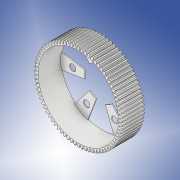
# Autodesk Inventor part: Flexspline
Saved by Autodesk Inventor 2017 SP1 (Build 210196100, 196)
## iProperties
Created: 2017-07-11
Part Number: Flexspline
Material: ABS Plastic
Document SubType Name: Modeling
Designer: zallen
Density: 1.06 g/cm^3
Appearance: CR White
Author: zallen
Autodesk Inventor part; units mm, degrees
ref_plane "YZ Plane" through (0, 0, 0) normal (1, 0, 0) x (0, 1, 0)
ref_plane "XZ Plane" through (0, 0, 0) normal (0, 1, 0) x (-1, 0, 0)
ref_plane "XY Plane" through (0, 0, 0) normal (0, 0, 1) x (1, 0, 0)
sketch "Sketch1" plane through (0, 0, 0) normal (0, 0, 1) x (1, 0, 0)
  circle A0 centre (0, 0) radius 44
  circle A1 centre (0, 0) radius 47 construction
  line L0 (0, 0) -> (52.2063, 0) construction
  arc A2 (46.9962, 0.6) -> (43.9777, 1.4) centre (41.6649, -13.4206) ccw
  arc A3 (46.9962, -0.6) -> (46.9962, 0.6) centre (27.0052, 0) ccw
  arc A4 (43.9777, -1.4) -> (46.9962, -0.6) centre (41.6649, 13.4206) ccw
  arc A5 (43.9777, -1.4) -> (43.9777, 1.4) centre (0, 0) ccw
  arc A6 (46.7861, 4.4789) -> (43.7119, 5.0269) centre (42.6309, -9.9341) ccw
  arc A7 (43.9431, 2.2364) -> (46.8852, 3.283) centre (40.4144, 16.8155) ccw
  arc A8 (46.8852, 3.283) -> (46.7861, 4.4789) centre (26.9129, 2.2301) ccw
  circle A9 centre (0, 0) radius 44
  arc A10 (43.9431, 2.2364) -> (43.7119, 5.0269) centre (0, 0) ccw
  arc A11 (46.2564, 8.3271) -> (43.1475, 8.6194) centre (43.3057, -6.3798) ccw
  arc A12 (43.6084, 5.8576) -> (46.454, 7.1435) centre (38.8877, 20.0954) ccw
  arc A13 (46.454, 7.1435) -> (46.2564, 8.3271) centre (26.6369, 4.4449) ccw
  circle A14 centre (0, 0) radius 44
  arc A15 (43.6084, 5.8576) -> (43.1475, 8.6194) centre (0, 0) ccw
  arc A16 (45.4108, 12.1185) -> (42.2883, 12.1531) centre (43.6846, -2.7818) ccw
  arc A17 (42.9757, 9.4387) -> (45.7054, 10.9552) centre (37.0954, 23.2381) ccw
  arc A18 (45.7054, 10.9552) -> (45.4108, 12.1185) centre (26.1788, 6.6294) ccw
  circle A19 centre (0, 0) radius 44
  arc A20 (42.9757, 9.4387) -> (42.2883, 12.1531) centre (0, 0) ccw
  arc A21 (44.255, 15.8271) -> (41.1403, 15.6037) centre (43.7651, 0.8351) ccw
  arc A22 (42.0495, 12.9554) -> (44.6446, 14.6921) centre (35.0498, 26.222) ccw
  arc A23 (44.6446, 14.6921) -> (44.255, 15.8271) centre (25.542, 8.7686) ccw
  circle A24 centre (0, 0) radius 44
  arc A25 (42.0495, 12.9554) -> (41.1403, 15.6037) centre (0, 0) ccw
  arc A26 (42.7968, 19.4276) -> (39.7113, 18.9477) centre (43.5467, 4.4464) ccw
  arc A27 (40.836, 16.3836) -> (43.2789, 18.3287) centre (32.7646, 29.0269) ccw
  arc A28 (43.2789, 18.3287) -> (42.7968, 19.4276) centre (24.7306, 10.8479) ccw
  circle A29 centre (0, 0) radius 44
  arc A30 (40.836, 16.3836) -> (39.7113, 18.9477) centre (0, 0) ccw
  arc A31 (41.0463, 22.8954) -> (38.0109, 22.1623) centre (43.0307, 8.0272) ccw
  arc A32 (39.3436, 19.6998) -> (41.6175, 21.84) centre (30.2557, 31.6334) ccw
  arc A33 (41.6175, 21.84) -> (41.0463, 22.8954) centre (23.7503, 12.853) ccw
  circle A34 centre (0, 0) radius 44
  arc A35 (39.3436, 19.6998) -> (38.0109, 22.1623) centre (0, 0) ccw
  arc A36 (39.0154, 26.2068) -> (36.0509, 25.2256) centre (42.2209, 11.5533) ccw
  arc A37 (37.5824, 22.8815) -> (39.6718, 25.2022) centre (27.5401, 34.0239) ccw
  arc A38 (39.6718, 25.2022) -> (39.0154, 26.2068) centre (22.6078, 14.7704) ccw
  circle A39 centre (0, 0) radius 44
  arc A40 (37.5824, 22.8815) -> (36.0509, 25.2256) centre (0, 0) ccw
  arc A41 (36.7181, 29.3391) -> (33.8447, 28.1165) centre (41.1226, 15.0004) ccw
  arc A42 (35.5645, 25.9069) -> (37.4551, 28.3922) centre (24.6364, 36.1819) ccw
  arc A43 (37.4551, 28.3922) -> (36.7181, 29.3391) centre (21.3109, 16.5869) ccw
  circle A44 centre (0, 0) radius 44
  arc A45 (35.5645, 25.9069) -> (33.8447, 28.1165) centre (0, 0) ccw
  arc A46 (34.1698, 32.2711) -> (31.4073, 30.8153) centre (39.7434, 18.345) ccw
  arc A47 (33.3037, 28.7553) -> (34.9826, 31.3882) centre (21.5644, 38.0928) ccw
  arc A48 (34.9826, 31.3882) -> (34.1698, 32.2711) centre (19.8684, 18.2901) ccw
  circle A49 centre (0, 0) radius 44
  arc A50 (33.3037, 28.7553) -> (31.4073, 30.8153) centre (0, 0) ccw
  arc A51 (31.3882, 34.9826) -> (28.7553, 33.3037) centre (38.0928, 21.5644) ccw
  arc A52 (30.8153, 31.4073) -> (32.2711, 34.1698) centre (18.345, 39.7434) ccw
  arc A53 (32.2711, 34.1698) -> (31.3882, 34.9826) centre (18.2901, 19.8684) ccw
  circle A54 centre (0, 0) radius 44
  arc A55 (30.8153, 31.4073) -> (28.7553, 33.3037) centre (0, 0) ccw
  arc A56 (28.3922, 37.4551) -> (25.9069, 35.5645) centre (36.1819, 24.6364) ccw
  arc A57 (28.1165, 33.8447) -> (29.3391, 36.7181) centre (15.0004, 41.1226) ccw
  arc A58 (29.3391, 36.7181) -> (28.3922, 37.4551) centre (16.5869, 21.3109) ccw
  circle A59 centre (0, 0) radius 44
  arc A60 (28.1165, 33.8447) -> (25.9069, 35.5645) centre (0, 0) ccw
  arc A61 (25.2022, 39.6718) -> (22.8815, 37.5824) centre (34.0239, 27.5401) ccw
  arc A62 (25.2256, 36.0509) -> (26.2068, 39.0154) centre (11.5533, 42.2209) ccw
  arc A63 (26.2068, 39.0154) -> (25.2022, 39.6718) centre (14.7704, 22.6078) ccw
  circle A64 centre (0, 0) radius 44
  arc A65 (25.2256, 36.0509) -> (22.8815, 37.5824) centre (0, 0) ccw
  arc A66 (21.84, 41.6175) -> (19.6998, 39.3436) centre (31.6334, 30.2557) ccw
  arc A67 (22.1623, 38.0109) -> (22.8954, 41.0463) centre (8.0272, 43.0307) ccw
  arc A68 (22.8954, 41.0463) -> (21.84, 41.6175) centre (12.853, 23.7503) ccw
  circle A69 centre (0, 0) radius 44
  arc A70 (22.1623, 38.0109) -> (19.6998, 39.3436) centre (0, 0) ccw
  arc A71 (18.3287, 43.2789) -> (16.3836, 40.836) centre (29.0269, 32.7646) ccw
  arc A72 (18.9477, 39.7113) -> (19.4276, 42.7968) centre (4.4464, 43.5467) ccw
  arc A73 (19.4276, 42.7968) -> (18.3287, 43.2789) centre (10.8479, 24.7306) ccw
  circle A74 centre (0, 0) radius 44
  arc A75 (18.9477, 39.7113) -> (16.3836, 40.836) centre (0, 0) ccw
  arc A76 (14.6921, 44.6446) -> (12.9554, 42.0495) centre (26.222, 35.0498) ccw
  arc A77 (15.6037, 41.1403) -> (15.8271, 44.255) centre (0.8351, 43.7651) ccw
  arc A78 (15.8271, 44.255) -> (14.6921, 44.6446) centre (8.7686, 25.542) ccw
  circle A79 centre (0, 0) radius 44
  arc A80 (15.6037, 41.1403) -> (12.9554, 42.0495) centre (0, 0) ccw
  arc A81 (10.9552, 45.7054) -> (9.4387, 42.9757) centre (23.2381, 37.0954) ccw
  arc A82 (12.1531, 42.2883) -> (12.1185, 45.4108) centre (-2.7818, 43.6846) ccw
  arc A83 (12.1185, 45.4108) -> (10.9552, 45.7054) centre (6.6294, 26.1788) ccw
  circle A84 centre (0, 0) radius 44
  arc A85 (12.1531, 42.2883) -> (9.4387, 42.9757) centre (0, 0) ccw
  arc A86 (7.1435, 46.454) -> (5.8576, 43.6084) centre (20.0954, 38.8877) ccw
  arc A87 (8.6194, 43.1475) -> (8.3271, 46.2564) centre (-6.3798, 43.3057) ccw
  arc A88 (8.3271, 46.2564) -> (7.1435, 46.454) centre (4.4449, 26.6369) ccw
  circle A89 centre (0, 0) radius 44
  arc A90 (8.6194, 43.1475) -> (5.8576, 43.6084) centre (0, 0) ccw
  arc A91 (3.283, 46.8852) -> (2.2364, 43.9431) centre (16.8155, 40.4144) ccw
  arc A92 (5.0269, 43.7119) -> (4.4789, 46.7861) centre (-9.9341, 42.6309) ccw
  arc A93 (4.4789, 46.7861) -> (3.283, 46.8852) centre (2.2301, 26.9129) ccw
  circle A94 centre (0, 0) radius 44
  arc A95 (5.0269, 43.7119) -> (2.2364, 43.9431) centre (0, 0) ccw
  arc A96 (-0.6, 46.9962) -> (-1.4, 43.9777) centre (13.4206, 41.6649) ccw
  arc A97 (1.4, 43.9777) -> (0.6, 46.9962) centre (-13.4206, 41.6649) ccw
  arc A98 (0.6, 46.9962) -> (-0.6, 46.9962) centre (0, 27.0052) ccw
  circle A99 centre (0, 0) radius 44
  arc A100 (1.4, 43.9777) -> (-1.4, 43.9777) centre (0, 0) ccw
  arc A101 (-4.4789, 46.7861) -> (-5.0269, 43.7119) centre (9.9341, 42.6309) ccw
  arc A102 (-2.2364, 43.9431) -> (-3.283, 46.8852) centre (-16.8155, 40.4144) ccw
  arc A103 (-3.283, 46.8852) -> (-4.4789, 46.7861) centre (-2.2301, 26.9129) ccw
  circle A104 centre (0, 0) radius 44
  arc A105 (-2.2364, 43.9431) -> (-5.0269, 43.7119) centre (0, 0) ccw
  arc A106 (-8.3271, 46.2564) -> (-8.6194, 43.1475) centre (6.3798, 43.3057) ccw
  arc A107 (-5.8576, 43.6084) -> (-7.1435, 46.454) centre (-20.0954, 38.8877) ccw
  arc A108 (-7.1435, 46.454) -> (-8.3271, 46.2564) centre (-4.4449, 26.6369) ccw
  circle A109 centre (0, 0) radius 44
  arc A110 (-5.8576, 43.6084) -> (-8.6194, 43.1475) centre (0, 0) ccw
  arc A111 (-12.1185, 45.4108) -> (-12.1531, 42.2883) centre (2.7818, 43.6846) ccw
  arc A112 (-9.4387, 42.9757) -> (-10.9552, 45.7054) centre (-23.2381, 37.0954) ccw
  arc A113 (-10.9552, 45.7054) -> (-12.1185, 45.4108) centre (-6.6294, 26.1788) ccw
  circle A114 centre (0, 0) radius 44
  arc A115 (-9.4387, 42.9757) -> (-12.1531, 42.2883) centre (0, 0) ccw
  arc A116 (-15.8271, 44.255) -> (-15.6037, 41.1403) centre (-0.8351, 43.7651) ccw
  arc A117 (-12.9554, 42.0495) -> (-14.6921, 44.6446) centre (-26.222, 35.0498) ccw
  arc A118 (-14.6921, 44.6446) -> (-15.8271, 44.255) centre (-8.7686, 25.542) ccw
  circle A119 centre (0, 0) radius 44
  arc A120 (-12.9554, 42.0495) -> (-15.6037, 41.1403) centre (0, 0) ccw
  arc A121 (-19.4276, 42.7968) -> (-18.9477, 39.7113) centre (-4.4464, 43.5467) ccw
  arc A122 (-16.3836, 40.836) -> (-18.3287, 43.2789) centre (-29.0269, 32.7646) ccw
  arc A123 (-18.3287, 43.2789) -> (-19.4276, 42.7968) centre (-10.8479, 24.7306) ccw
  circle A124 centre (0, 0) radius 44
  arc A125 (-16.3836, 40.836) -> (-18.9477, 39.7113) centre (0, 0) ccw
  arc A126 (-22.8954, 41.0463) -> (-22.1623, 38.0109) centre (-8.0272, 43.0307) ccw
  arc A127 (-19.6998, 39.3436) -> (-21.84, 41.6175) centre (-31.6334, 30.2557) ccw
  arc A128 (-21.84, 41.6175) -> (-22.8954, 41.0463) centre (-12.853, 23.7503) ccw
  circle A129 centre (0, 0) radius 44
  arc A130 (-19.6998, 39.3436) -> (-22.1623, 38.0109) centre (0, 0) ccw
  arc A131 (-26.2068, 39.0154) -> (-25.2256, 36.0509) centre (-11.5533, 42.2209) ccw
  arc A132 (-22.8815, 37.5824) -> (-25.2022, 39.6718) centre (-34.0239, 27.5401) ccw
  arc A133 (-25.2022, 39.6718) -> (-26.2068, 39.0154) centre (-14.7704, 22.6078) ccw
  circle A134 centre (0, 0) radius 44
  arc A135 (-22.8815, 37.5824) -> (-25.2256, 36.0509) centre (0, 0) ccw
  arc A136 (-29.3391, 36.7181) -> (-28.1165, 33.8447) centre (-15.0004, 41.1226) ccw
  arc A137 (-25.9069, 35.5645) -> (-28.3922, 37.4551) centre (-36.1819, 24.6364) ccw
  arc A138 (-28.3922, 37.4551) -> (-29.3391, 36.7181) centre (-16.5869, 21.3109) ccw
  circle A139 centre (0, 0) radius 44
  arc A140 (-25.9069, 35.5645) -> (-28.1165, 33.8447) centre (0, 0) ccw
  arc A141 (-32.2711, 34.1698) -> (-30.8153, 31.4073) centre (-18.345, 39.7434) ccw
  arc A142 (-28.7553, 33.3037) -> (-31.3882, 34.9826) centre (-38.0928, 21.5644) ccw
  arc A143 (-31.3882, 34.9826) -> (-32.2711, 34.1698) centre (-18.2901, 19.8684) ccw
  circle A144 centre (0, 0) radius 44
  arc A145 (-28.7553, 33.3037) -> (-30.8153, 31.4073) centre (0, 0) ccw
  arc A146 (-34.9826, 31.3882) -> (-33.3037, 28.7553) centre (-21.5644, 38.0928) ccw
  arc A147 (-31.4073, 30.8153) -> (-34.1698, 32.2711) centre (-39.7434, 18.345) ccw
  arc A148 (-34.1698, 32.2711) -> (-34.9826, 31.3882) centre (-19.8684, 18.2901) ccw
  circle A149 centre (0, 0) radius 44
  arc A150 (-31.4073, 30.8153) -> (-33.3037, 28.7553) centre (0, 0) ccw
  arc A151 (-37.4551, 28.3922) -> (-35.5645, 25.9069) centre (-24.6364, 36.1819) ccw
  arc A152 (-33.8447, 28.1165) -> (-36.7181, 29.3391) centre (-41.1226, 15.0004) ccw
  arc A153 (-36.7181, 29.3391) -> (-37.4551, 28.3922) centre (-21.3109, 16.5869) ccw
  circle A154 centre (0, 0) radius 44
  arc A155 (-33.8447, 28.1165) -> (-35.5645, 25.9069) centre (0, 0) ccw
  arc A156 (-39.6718, 25.2022) -> (-37.5824, 22.8815) centre (-27.5401, 34.0239) ccw
  arc A157 (-36.0509, 25.2256) -> (-39.0154, 26.2068) centre (-42.2209, 11.5533) ccw
  arc A158 (-39.0154, 26.2068) -> (-39.6718, 25.2022) centre (-22.6078, 14.7704) ccw
  circle A159 centre (0, 0) radius 44
  arc A160 (-36.0509, 25.2256) -> (-37.5824, 22.8815) centre (0, 0) ccw
  arc A161 (-41.6175, 21.84) -> (-39.3436, 19.6998) centre (-30.2557, 31.6334) ccw
  arc A162 (-38.0109, 22.1623) -> (-41.0463, 22.8954) centre (-43.0307, 8.0272) ccw
  arc A163 (-41.0463, 22.8954) -> (-41.6175, 21.84) centre (-23.7503, 12.853) ccw
  circle A164 centre (0, 0) radius 44
  arc A165 (-38.0109, 22.1623) -> (-39.3436, 19.6998) centre (0, 0) ccw
  arc A166 (-43.2789, 18.3287) -> (-40.836, 16.3836) centre (-32.7646, 29.0269) ccw
  arc A167 (-39.7113, 18.9477) -> (-42.7968, 19.4276) centre (-43.5467, 4.4464) ccw
  arc A168 (-42.7968, 19.4276) -> (-43.2789, 18.3287) centre (-24.7306, 10.8479) ccw
  circle A169 centre (0, 0) radius 44
  arc A170 (-39.7113, 18.9477) -> (-40.836, 16.3836) centre (0, 0) ccw
  arc A171 (-44.6446, 14.6921) -> (-42.0495, 12.9554) centre (-35.0498, 26.222) ccw
  arc A172 (-41.1403, 15.6037) -> (-44.255, 15.8271) centre (-43.7651, 0.8351) ccw
  arc A173 (-44.255, 15.8271) -> (-44.6446, 14.6921) centre (-25.542, 8.7686) ccw
  circle A174 centre (0, 0) radius 44
  arc A175 (-41.1403, 15.6037) -> (-42.0495, 12.9554) centre (0, 0) ccw
  arc A176 (-45.7054, 10.9552) -> (-42.9757, 9.4387) centre (-37.0954, 23.2381) ccw
  arc A177 (-42.2883, 12.1531) -> (-45.4108, 12.1185) centre (-43.6846, -2.7818) ccw
  arc A178 (-45.4108, 12.1185) -> (-45.7054, 10.9552) centre (-26.1788, 6.6294) ccw
  circle A179 centre (0, 0) radius 44
  arc A180 (-42.2883, 12.1531) -> (-42.9757, 9.4387) centre (0, 0) ccw
  arc A181 (-46.454, 7.1435) -> (-43.6084, 5.8576) centre (-38.8877, 20.0954) ccw
  arc A182 (-43.1475, 8.6194) -> (-46.2564, 8.3271) centre (-43.3057, -6.3798) ccw
  arc A183 (-46.2564, 8.3271) -> (-46.454, 7.1435) centre (-26.6369, 4.4449) ccw
  circle A184 centre (0, 0) radius 44
  arc A185 (-43.1475, 8.6194) -> (-43.6084, 5.8576) centre (0, 0) ccw
  arc A186 (-46.8852, 3.283) -> (-43.9431, 2.2364) centre (-40.4144, 16.8155) ccw
  arc A187 (-43.7119, 5.0269) -> (-46.7861, 4.4789) centre (-42.6309, -9.9341) ccw
  arc A188 (-46.7861, 4.4789) -> (-46.8852, 3.283) centre (-26.9129, 2.2301) ccw
  circle A189 centre (0, 0) radius 44
  arc A190 (-43.7119, 5.0269) -> (-43.9431, 2.2364) centre (0, 0) ccw
  arc A191 (-46.9962, -0.6) -> (-43.9777, -1.4) centre (-41.6649, 13.4206) ccw
  arc A192 (-43.9777, 1.4) -> (-46.9962, 0.6) centre (-41.6649, -13.4206) ccw
  arc A193 (-46.9962, 0.6) -> (-46.9962, -0.6) centre (-27.0052, 0) ccw
  circle A194 centre (0, 0) radius 44
  arc A195 (-43.9777, 1.4) -> (-43.9777, -1.4) centre (0, 0) ccw
  arc A196 (-46.7861, -4.4789) -> (-43.7119, -5.0269) centre (-42.6309, 9.9341) ccw
  arc A197 (-43.9431, -2.2364) -> (-46.8852, -3.283) centre (-40.4144, -16.8155) ccw
  arc A198 (-46.8852, -3.283) -> (-46.7861, -4.4789) centre (-26.9129, -2.2301) ccw
  circle A199 centre (0, 0) radius 44
  arc A200 (-43.9431, -2.2364) -> (-43.7119, -5.0269) centre (0, 0) ccw
  arc A201 (-46.2564, -8.3271) -> (-43.1475, -8.6194) centre (-43.3057, 6.3798) ccw
  arc A202 (-43.6084, -5.8576) -> (-46.454, -7.1435) centre (-38.8877, -20.0954) ccw
  arc A203 (-46.454, -7.1435) -> (-46.2564, -8.3271) centre (-26.6369, -4.4449) ccw
  circle A204 centre (0, 0) radius 44
  arc A205 (-43.6084, -5.8576) -> (-43.1475, -8.6194) centre (0, 0) ccw
  arc A206 (-45.4108, -12.1185) -> (-42.2883, -12.1531) centre (-43.6846, 2.7818) ccw
  arc A207 (-42.9757, -9.4387) -> (-45.7054, -10.9552) centre (-37.0954, -23.2381) ccw
  arc A208 (-45.7054, -10.9552) -> (-45.4108, -12.1185) centre (-26.1788, -6.6294) ccw
  circle A209 centre (0, 0) radius 44
  arc A210 (-42.9757, -9.4387) -> (-42.2883, -12.1531) centre (0, 0) ccw
  arc A211 (-44.255, -15.8271) -> (-41.1403, -15.6037) centre (-43.7651, -0.8351) ccw
  arc A212 (-42.0495, -12.9554) -> (-44.6446, -14.6921) centre (-35.0498, -26.222) ccw
  arc A213 (-44.6446, -14.6921) -> (-44.255, -15.8271) centre (-25.542, -8.7686) ccw
  circle A214 centre (0, 0) radius 44
  arc A215 (-42.0495, -12.9554) -> (-41.1403, -15.6037) centre (0, 0) ccw
  arc A216 (-42.7968, -19.4276) -> (-39.7113, -18.9477) centre (-43.5467, -4.4464) ccw
  arc A217 (-40.836, -16.3836) -> (-43.2789, -18.3287) centre (-32.7646, -29.0269) ccw
  arc A218 (-43.2789, -18.3287) -> (-42.7968, -19.4276) centre (-24.7306, -10.8479) ccw
  circle A219 centre (0, 0) radius 44
  arc A220 (-40.836, -16.3836) -> (-39.7113, -18.9477) centre (0, 0) ccw
  arc A221 (-41.0463, -22.8954) -> (-38.0109, -22.1623) centre (-43.0307, -8.0272) ccw
  arc A222 (-39.3436, -19.6998) -> (-41.6175, -21.84) centre (-30.2557, -31.6334) ccw
  arc A223 (-41.6175, -21.84) -> (-41.0463, -22.8954) centre (-23.7503, -12.853) ccw
  circle A224 centre (0, 0) radius 44
  arc A225 (-39.3436, -19.6998) -> (-38.0109, -22.1623) centre (0, 0) ccw
  arc A226 (-39.0154, -26.2068) -> (-36.0509, -25.2256) centre (-42.2209, -11.5533) ccw
  arc A227 (-37.5824, -22.8815) -> (-39.6718, -25.2022) centre (-27.5401, -34.0239) ccw
  arc A228 (-39.6718, -25.2022) -> (-39.0154, -26.2068) centre (-22.6078, -14.7704) ccw
  circle A229 centre (0, 0) radius 44
  arc A230 (-37.5824, -22.8815) -> (-36.0509, -25.2256) centre (0, 0) ccw
  arc A231 (-36.7181, -29.3391) -> (-33.8447, -28.1165) centre (-41.1226, -15.0004) ccw
  arc A232 (-35.5645, -25.9069) -> (-37.4551, -28.3922) centre (-24.6364, -36.1819) ccw
  arc A233 (-37.4551, -28.3922) -> (-36.7181, -29.3391) centre (-21.3109, -16.5869) ccw
  circle A234 centre (0, 0) radius 44
  arc A235 (-35.5645, -25.9069) -> (-33.8447, -28.1165) centre (0, 0) ccw
  arc A236 (-34.1698, -32.2711) -> (-31.4073, -30.8153) centre (-39.7434, -18.345) ccw
  arc A237 (-33.3037, -28.7553) -> (-34.9826, -31.3882) centre (-21.5644, -38.0928) ccw
  arc A238 (-34.9826, -31.3882) -> (-34.1698, -32.2711) centre (-19.8684, -18.2901) ccw
  circle A239 centre (0, 0) radius 44
  arc A240 (-33.3037, -28.7553) -> (-31.4073, -30.8153) centre (0, 0) ccw
  arc A241 (-31.3882, -34.9826) -> (-28.7553, -33.3037) centre (-38.0928, -21.5644) ccw
  arc A242 (-30.8153, -31.4073) -> (-32.2711, -34.1698) centre (-18.345, -39.7434) ccw
  arc A243 (-32.2711, -34.1698) -> (-31.3882, -34.9826) centre (-18.2901, -19.8684) ccw
  circle A244 centre (0, 0) radius 44
  arc A245 (-30.8153, -31.4073) -> (-28.7553, -33.3037) centre (0, 0) ccw
  arc A246 (-28.3922, -37.4551) -> (-25.9069, -35.5645) centre (-36.1819, -24.6364) ccw
  arc A247 (-28.1165, -33.8447) -> (-29.3391, -36.7181) centre (-15.0004, -41.1226) ccw
  arc A248 (-29.3391, -36.7181) -> (-28.3922, -37.4551) centre (-16.5869, -21.3109) ccw
  circle A249 centre (0, 0) radius 44
  arc A250 (-28.1165, -33.8447) -> (-25.9069, -35.5645) centre (0, 0) ccw
  arc A251 (-25.2022, -39.6718) -> (-22.8815, -37.5824) centre (-34.0239, -27.5401) ccw
  arc A252 (-25.2256, -36.0509) -> (-26.2068, -39.0154) centre (-11.5533, -42.2209) ccw
  arc A253 (-26.2068, -39.0154) -> (-25.2022, -39.6718) centre (-14.7704, -22.6078) ccw
  circle A254 centre (0, 0) radius 44
  arc A255 (-25.2256, -36.0509) -> (-22.8815, -37.5824) centre (0, 0) ccw
  arc A256 (-21.84, -41.6175) -> (-19.6998, -39.3436) centre (-31.6334, -30.2557) ccw
  arc A257 (-22.1623, -38.0109) -> (-22.8954, -41.0463) centre (-8.0272, -43.0307) ccw
  arc A258 (-22.8954, -41.0463) -> (-21.84, -41.6175) centre (-12.853, -23.7503) ccw
  circle A259 centre (0, 0) radius 44
  arc A260 (-22.1623, -38.0109) -> (-19.6998, -39.3436) centre (0, 0) ccw
  arc A261 (-18.3287, -43.2789) -> (-16.3836, -40.836) centre (-29.0269, -32.7646) ccw
  arc A262 (-18.9477, -39.7113) -> (-19.4276, -42.7968) centre (-4.4464, -43.5467) ccw
  arc A263 (-19.4276, -42.7968) -> (-18.3287, -43.2789) centre (-10.8479, -24.7306) ccw
  circle A264 centre (0, 0) radius 44
  arc A265 (-18.9477, -39.7113) -> (-16.3836, -40.836) centre (0, 0) ccw
  arc A266 (-14.6921, -44.6446) -> (-12.9554, -42.0495) centre (-26.222, -35.0498) ccw
  arc A267 (-15.6037, -41.1403) -> (-15.8271, -44.255) centre (-0.8351, -43.7651) ccw
  arc A268 (-15.8271, -44.255) -> (-14.6921, -44.6446) centre (-8.7686, -25.542) ccw
  circle A269 centre (0, 0) radius 44
  arc A270 (-15.6037, -41.1403) -> (-12.9554, -42.0495) centre (0, 0) ccw
  arc A271 (-10.9552, -45.7054) -> (-9.4387, -42.9757) centre (-23.2381, -37.0954) ccw
  arc A272 (-12.1531, -42.2883) -> (-12.1185, -45.4108) centre (2.7818, -43.6846) ccw
  arc A273 (-12.1185, -45.4108) -> (-10.9552, -45.7054) centre (-6.6294, -26.1788) ccw
  circle A274 centre (0, 0) radius 44
  arc A275 (-12.1531, -42.2883) -> (-9.4387, -42.9757) centre (0, 0) ccw
  arc A276 (-7.1435, -46.454) -> (-5.8576, -43.6084) centre (-20.0954, -38.8877) ccw
  arc A277 (-8.6194, -43.1475) -> (-8.3271, -46.2564) centre (6.3798, -43.3057) ccw
  arc A278 (-8.3271, -46.2564) -> (-7.1435, -46.454) centre (-4.4449, -26.6369) ccw
  circle A279 centre (0, 0) radius 44
  arc A280 (-8.6194, -43.1475) -> (-5.8576, -43.6084) centre (0, 0) ccw
  arc A281 (-3.283, -46.8852) -> (-2.2364, -43.9431) centre (-16.8155, -40.4144) ccw
  arc A282 (-5.0269, -43.7119) -> (-4.4789, -46.7861) centre (9.9341, -42.6309) ccw
  arc A283 (-4.4789, -46.7861) -> (-3.283, -46.8852) centre (-2.2301, -26.9129) ccw
  circle A284 centre (0, 0) radius 44
  arc A285 (-5.0269, -43.7119) -> (-2.2364, -43.9431) centre (0, 0) ccw
  arc A286 (0.6, -46.9962) -> (1.4, -43.9777) centre (-13.4206, -41.6649) ccw
  arc A287 (-1.4, -43.9777) -> (-0.6, -46.9962) centre (13.4206, -41.6649) ccw
  arc A288 (-0.6, -46.9962) -> (0.6, -46.9962) centre (0, -27.0052) ccw
  circle A289 centre (0, 0) radius 44
  arc A290 (-1.4, -43.9777) -> (1.4, -43.9777) centre (0, 0) ccw
  arc A291 (4.4789, -46.7861) -> (5.0269, -43.7119) centre (-9.9341, -42.6309) ccw
  arc A292 (2.2364, -43.9431) -> (3.283, -46.8852) centre (16.8155, -40.4144) ccw
  arc A293 (3.283, -46.8852) -> (4.4789, -46.7861) centre (2.2301, -26.9129) ccw
  circle A294 centre (0, 0) radius 44
  arc A295 (2.2364, -43.9431) -> (5.0269, -43.7119) centre (0, 0) ccw
  arc A296 (8.3271, -46.2564) -> (8.6194, -43.1475) centre (-6.3798, -43.3057) ccw
  arc A297 (5.8576, -43.6084) -> (7.1435, -46.454) centre (20.0954, -38.8877) ccw
  arc A298 (7.1435, -46.454) -> (8.3271, -46.2564) centre (4.4449, -26.6369) ccw
  circle A299 centre (0, 0) radius 44
  arc A300 (5.8576, -43.6084) -> (8.6194, -43.1475) centre (0, 0) ccw
  arc A301 (12.1185, -45.4108) -> (12.1531, -42.2883) centre (-2.7818, -43.6846) ccw
  arc A302 (9.4387, -42.9757) -> (10.9552, -45.7054) centre (23.2381, -37.0954) ccw
  arc A303 (10.9552, -45.7054) -> (12.1185, -45.4108) centre (6.6294, -26.1788) ccw
  circle A304 centre (0, 0) radius 44
  arc A305 (9.4387, -42.9757) -> (12.1531, -42.2883) centre (0, 0) ccw
  arc A306 (15.8271, -44.255) -> (15.6037, -41.1403) centre (0.8351, -43.7651) ccw
  arc A307 (12.9554, -42.0495) -> (14.6921, -44.6446) centre (26.222, -35.0498) ccw
  arc A308 (14.6921, -44.6446) -> (15.8271, -44.255) centre (8.7686, -25.542) ccw
  circle A309 centre (0, 0) radius 44
  arc A310 (12.9554, -42.0495) -> (15.6037, -41.1403) centre (0, 0) ccw
  arc A311 (19.4276, -42.7968) -> (18.9477, -39.7113) centre (4.4464, -43.5467) ccw
  arc A312 (16.3836, -40.836) -> (18.3287, -43.2789) centre (29.0269, -32.7646) ccw
  arc A313 (18.3287, -43.2789) -> (19.4276, -42.7968) centre (10.8479, -24.7306) ccw
  circle A314 centre (0, 0) radius 44
  arc A315 (16.3836, -40.836) -> (18.9477, -39.7113) centre (0, 0) ccw
  arc A316 (22.8954, -41.0463) -> (22.1623, -38.0109) centre (8.0272, -43.0307) ccw
  arc A317 (19.6998, -39.3436) -> (21.84, -41.6175) centre (31.6334, -30.2557) ccw
  arc A318 (21.84, -41.6175) -> (22.8954, -41.0463) centre (12.853, -23.7503) ccw
  circle A319 centre (0, 0) radius 44
  arc A320 (19.6998, -39.3436) -> (22.1623, -38.0109) centre (0, 0) ccw
  arc A321 (26.2068, -39.0154) -> (25.2256, -36.0509) centre (11.5533, -42.2209) ccw
  arc A322 (22.8815, -37.5824) -> (25.2022, -39.6718) centre (34.0239, -27.5401) ccw
  arc A323 (25.2022, -39.6718) -> (26.2068, -39.0154) centre (14.7704, -22.6078) ccw
  circle A324 centre (0, 0) radius 44
  arc A325 (22.8815, -37.5824) -> (25.2256, -36.0509) centre (0, 0) ccw
  arc A326 (29.3391, -36.7181) -> (28.1165, -33.8447) centre (15.0004, -41.1226) ccw
  arc A327 (25.9069, -35.5645) -> (28.3922, -37.4551) centre (36.1819, -24.6364) ccw
  arc A328 (28.3922, -37.4551) -> (29.3391, -36.7181) centre (16.5869, -21.3109) ccw
  circle A329 centre (0, 0) radius 44
  arc A330 (25.9069, -35.5645) -> (28.1165, -33.8447) centre (0, 0) ccw
  arc A331 (32.2711, -34.1698) -> (30.8153, -31.4073) centre (18.345, -39.7434) ccw
  arc A332 (28.7553, -33.3037) -> (31.3882, -34.9826) centre (38.0928, -21.5644) ccw
  arc A333 (31.3882, -34.9826) -> (32.2711, -34.1698) centre (18.2901, -19.8684) ccw
  circle A334 centre (0, 0) radius 44
  arc A335 (28.7553, -33.3037) -> (30.8153, -31.4073) centre (0, 0) ccw
  arc A336 (34.9826, -31.3882) -> (33.3037, -28.7553) centre (21.5644, -38.0928) ccw
  arc A337 (31.4073, -30.8153) -> (34.1698, -32.2711) centre (39.7434, -18.345) ccw
  arc A338 (34.1698, -32.2711) -> (34.9826, -31.3882) centre (19.8684, -18.2901) ccw
  circle A339 centre (0, 0) radius 44
  arc A340 (31.4073, -30.8153) -> (33.3037, -28.7553) centre (0, 0) ccw
  arc A341 (37.4551, -28.3922) -> (35.5645, -25.9069) centre (24.6364, -36.1819) ccw
  arc A342 (33.8447, -28.1165) -> (36.7181, -29.3391) centre (41.1226, -15.0004) ccw
  arc A343 (36.7181, -29.3391) -> (37.4551, -28.3922) centre (21.3109, -16.5869) ccw
  circle A344 centre (0, 0) radius 44
  arc A345 (33.8447, -28.1165) -> (35.5645, -25.9069) centre (0, 0) ccw
  arc A346 (39.6718, -25.2022) -> (37.5824, -22.8815) centre (27.5401, -34.0239) ccw
  arc A347 (36.0509, -25.2256) -> (39.0154, -26.2068) centre (42.2209, -11.5533) ccw
  arc A348 (39.0154, -26.2068) -> (39.6718, -25.2022) centre (22.6078, -14.7704) ccw
  circle A349 centre (0, 0) radius 44
  arc A350 (36.0509, -25.2256) -> (37.5824, -22.8815) centre (0, 0) ccw
  arc A351 (41.6175, -21.84) -> (39.3436, -19.6998) centre (30.2557, -31.6334) ccw
  arc A352 (38.0109, -22.1623) -> (41.0463, -22.8954) centre (43.0307, -8.0272) ccw
  arc A353 (41.0463, -22.8954) -> (41.6175, -21.84) centre (23.7503, -12.853) ccw
  circle A354 centre (0, 0) radius 44
  arc A355 (38.0109, -22.1623) -> (39.3436, -19.6998) centre (0, 0) ccw
  arc A356 (43.2789, -18.3287) -> (40.836, -16.3836) centre (32.7646, -29.0269) ccw
  arc A357 (39.7113, -18.9477) -> (42.7968, -19.4276) centre (43.5467, -4.4464) ccw
  arc A358 (42.7968, -19.4276) -> (43.2789, -18.3287) centre (24.7306, -10.8479) ccw
  circle A359 centre (0, 0) radius 44
  arc A360 (39.7113, -18.9477) -> (40.836, -16.3836) centre (0, 0) ccw
  arc A361 (44.6446, -14.6921) -> (42.0495, -12.9554) centre (35.0498, -26.222) ccw
  arc A362 (41.1403, -15.6037) -> (44.255, -15.8271) centre (43.7651, -0.8351) ccw
  arc A363 (44.255, -15.8271) -> (44.6446, -14.6921) centre (25.542, -8.7686) ccw
  circle A364 centre (0, 0) radius 44
  arc A365 (41.1403, -15.6037) -> (42.0495, -12.9554) centre (0, 0) ccw
  arc A366 (45.7054, -10.9552) -> (42.9757, -9.4387) centre (37.0954, -23.2381) ccw
  arc A367 (42.2883, -12.1531) -> (45.4108, -12.1185) centre (43.6846, 2.7818) ccw
  arc A368 (45.4108, -12.1185) -> (45.7054, -10.9552) centre (26.1788, -6.6294) ccw
  circle A369 centre (0, 0) radius 44
  arc A370 (42.2883, -12.1531) -> (42.9757, -9.4387) centre (0, 0) ccw
  arc A371 (46.454, -7.1435) -> (43.6084, -5.8576) centre (38.8877, -20.0954) ccw
  arc A372 (43.1475, -8.6194) -> (46.2564, -8.3271) centre (43.3057, 6.3798) ccw
  arc A373 (46.2564, -8.3271) -> (46.454, -7.1435) centre (26.6369, -4.4449) ccw
  circle A374 centre (0, 0) radius 44
  arc A375 (43.1475, -8.6194) -> (43.6084, -5.8576) centre (0, 0) ccw
  arc A376 (46.8852, -3.283) -> (43.9431, -2.2364) centre (40.4144, -16.8155) ccw
  arc A377 (43.7119, -5.0269) -> (46.7861, -4.4789) centre (42.6309, 9.9341) ccw
  arc A378 (46.7861, -4.4789) -> (46.8852, -3.283) centre (26.9129, -2.2301) ccw
  circle A379 centre (0, 0) radius 44
  arc A380 (43.7119, -5.0269) -> (43.9431, -2.2364) centre (0, 0) ccw
  point P0 (47.0052, 0)
  point P1 (46.8446, 3.8817)
  point P2 (46.3641, 7.7368)
  point P3 (45.5668, 11.5391)
  point P4 (44.4583, 15.2626)
  point P5 (43.0461, 18.8818)
  point P6 (41.3398, 22.372)
  point P7 (39.3512, 25.7094)
  point P8 (37.0937, 28.8712)
  point P9 (34.5828, 31.8357)
  point P10 (31.8357, 34.5828)
  point P11 (28.8712, 37.0937)
  point P12 (25.7094, 39.3512)
  point P13 (22.372, 41.3398)
  point P14 (18.8818, 43.0461)
  point P15 (15.2626, 44.4583)
  point P16 (11.5391, 45.5668)
  point P17 (7.7368, 46.3641)
  point P18 (3.8817, 46.8446)
  point P19 (0, 47.0052)
  point P20 (-3.8817, 46.8446)
  point P21 (-7.7368, 46.3641)
  point P22 (-11.5391, 45.5668)
  point P23 (-15.2626, 44.4583)
  point P24 (-18.8818, 43.0461)
  point P25 (-22.372, 41.3398)
  point P26 (-25.7094, 39.3512)
  point P27 (-28.8712, 37.0937)
  point P28 (-31.8357, 34.5828)
  point P29 (-34.5828, 31.8357)
  point P30 (-37.0937, 28.8712)
  point P31 (-39.3512, 25.7094)
  point P32 (-41.3398, 22.372)
  point P33 (-43.0461, 18.8818)
  point P34 (-44.4583, 15.2626)
  point P35 (-45.5668, 11.5391)
  point P36 (-46.3641, 7.7368)
  point P37 (-46.8446, 3.8817)
  point P38 (-47.0052, 0)
  point P39 (-46.8446, -3.8817)
  point P40 (-46.3641, -7.7368)
  point P41 (-45.5668, -11.5391)
  point P42 (-44.4583, -15.2626)
  point P43 (-43.0461, -18.8818)
  point P44 (-41.3398, -22.372)
  point P45 (-39.3512, -25.7094)
  point P46 (-37.0937, -28.8712)
  point P47 (-34.5828, -31.8357)
  point P48 (-31.8357, -34.5828)
  point P49 (-28.8712, -37.0937)
  point P50 (-25.7094, -39.3512)
  point P51 (-22.372, -41.3398)
  point P52 (-18.8818, -43.0461)
  point P53 (-15.2626, -44.4583)
  point P54 (-11.5391, -45.5668)
  point P55 (-7.7368, -46.3641)
  point P56 (-3.8817, -46.8446)
  point P57 (0, -47.0052)
  point P58 (3.8817, -46.8446)
  point P59 (7.7368, -46.3641)
  point P60 (11.5391, -45.5668)
  point P61 (15.2626, -44.4583)
  point P62 (18.8818, -43.0461)
  point P63 (22.372, -41.3398)
  point P64 (25.7094, -39.3512)
  point P65 (28.8712, -37.0937)
  point P66 (31.8357, -34.5828)
  point P67 (34.5828, -31.8357)
  point P68 (37.0937, -28.8712)
  point P69 (39.3512, -25.7094)
  point P70 (41.3398, -22.372)
  point P71 (43.0461, -18.8818)
  point P72 (44.4583, -15.2626)
  point P73 (45.5668, -11.5391)
  point P74 (46.3641, -7.7368)
  point P75 (46.8446, -3.8817)
  dimension "d2" = 15
  dimension "d3" = 20
  dimension "d4" = 1.2
  dimension "d5" = 1.4
  dimension "d6" = 3
  dimension "d9" = 360
  constraints: 611 point on circle, 305 centre point, 2 coincident, 2 end point, 2 symmetric about line, 1 horizontal, 1 point on line, 1446 other
  measures "d2" radius of A2
  measures "d3" radius of A3
  measures "d4" distance of A1.end A1.start
  measures "d5" distance from line of L0 A2.end
extrude "Extrusion1" add sketch "Sketch1" along normal blind 24
sketch "Sketch2" plane through (0, 0, 24) normal (0, 0, 1) x (1, 0, 0)
  circle A0 centre (0, 0) radius 43
  dimension "d13" = 86
  constraints: 1 centre point, 1 coincident
  measures "d13" diameter of A0
extrude "Extrusion2" cut sketch "Sketch2" against normal through all
sketch "Sketch3" plane through (0, 0, 0) normal (0, 0, -1) x (-1, 0, 0)
  circle A0 centre (0, 0) radius 11
  circle A1 centre (0, 0) radius 17.5 construction
  circle A2 centre (0, 0) radius 43 construction
  line L0 (-14, 40.6571) -> (-5, 16.7705)
  line L1 (14, 40.6571) -> (5, 16.7705)
  arc A3 (14, 40.6571) -> (-14, 40.6571) centre (0, 0) ccw
  arc A4 (5, 16.7705) -> (-5, 16.7705) centre (0, 0) ccw
  circle A5 centre (0, 0) radius 30 construction
  line L2 (9.4137, 28.4848) -> (19.9617, 22.3949) construction
  line L3 (14.6877, 25.4398) -> (15, 25.9808) construction
  circle A6 centre (15, 25.9808) radius 3.5
  circle A7 centre (-15, 25.9808) radius 3.5
  circle A8 centre (-30, 0) radius 3.5
  circle A9 centre (-15, -25.9808) radius 3.5
  circle A10 centre (15, -25.9808) radius 3.5
  circle A11 centre (30, 0) radius 3.5
  arc A12 (-28.2101, 32.4529) -> (-42.2101, 8.2042) centre (0, 0) ccw
  line L4 (-28.2101, 32.4529) -> (-12.0237, 12.7154)
  line L5 (-42.2101, 8.2042) -> (-17.0237, 4.0551)
  arc A13 (-12.0237, 12.7154) -> (-17.0237, 4.0551) centre (0, 0) ccw
  arc A14 (-42.2101, -8.2042) -> (-28.2101, -32.4529) centre (0, 0) ccw
  line L6 (-42.2101, -8.2042) -> (-17.0237, -4.0551)
  line L7 (-28.2101, -32.4529) -> (-12.0237, -12.7154)
  arc A15 (-17.0237, -4.0551) -> (-12.0237, -12.7154) centre (0, 0) ccw
  arc A16 (-14, -40.6571) -> (14, -40.6571) centre (0, 0) ccw
  line L8 (-14, -40.6571) -> (-5, -16.7705)
  line L9 (14, -40.6571) -> (5, -16.7705)
  arc A17 (-5, -16.7705) -> (5, -16.7705) centre (0, 0) ccw
  arc A18 (28.2101, -32.4529) -> (42.2101, -8.2042) centre (0, 0) ccw
  line L10 (28.2101, -32.4529) -> (12.0237, -12.7154)
  line L11 (42.2101, -8.2042) -> (17.0237, -4.0551)
  arc A19 (12.0237, -12.7154) -> (17.0237, -4.0551) centre (0, 0) ccw
  arc A20 (42.2101, 8.2042) -> (28.2101, 32.4529) centre (0, 0) ccw
  line L12 (42.2101, 8.2042) -> (17.0237, 4.0551)
  line L13 (28.2101, 32.4529) -> (12.0237, 12.7154)
  arc A21 (17.0237, 4.0551) -> (12.0237, 12.7154) centre (0, 0) ccw
  circle A22 centre (0, 0) radius 44
  point P0 (-19.9617, 22.3949)
  point P1 (-29.3754, -6.0899)
  point P2 (-9.4137, -28.4848)
  point P3 (19.9617, -22.3949)
  point P4 (29.3754, 6.0899)
  dimension "d16" = 22
  dimension "d17" = 35
  dimension "d18" = 86
  dimension "d20" = 14
  dimension "d21" = 5
  dimension "d22" = 14
  dimension "d23" = 5
  dimension "d28" = 60
  dimension "d29" = 7
  dimension "d32" = 360
  dimension "d38" = 360
  dimension "d44" = 88
  constraints: 31 point on circle, 28 end point, 23 centre point, 7 point on line, 5 coincident, 3 concentric, 1 midpoint, 1 perpendicular, 80 other
  measures "d16" diameter of A0
  measures "d17" diameter of A1
  measures "d18" diameter of A2
  measures "d20" horizontal distance of point (0, 0) L0.start
  measures "d21" horizontal distance of point (0, 0) L0.end
  measures "d22" horizontal distance of point (0, 0) L1.start
  measures "d23" horizontal distance of point (0, 0) L1.end
  measures "d28" diameter of A5
  measures "d29" diameter of A6
  measures "d44" diameter of A22
extrude "Extrusion4" add sketch "Sketch3" along normal blind 1
sketch "Sketch4" plane through (0, 0, -1) normal (0, 0, -1) x (-1, 0, 0)
  circle A0 centre (0, 0) radius 17.5
  arc A1 (-12.0237, 12.7154) -> (-17.0237, 4.0551) centre (0, 0) ccw
  line L0 (0, 0) -> (-15.1554, 8.75) construction
  arc A2 (-12.0237, 12.7154) -> (-17.0237, 4.0551) centre (0, 0) ccw
  constraints: 7 point on circle, 2 centre point, 2 end point, 1 coincident, 4 other
extrude "Extrusion5" cut sketch "Sketch4" against normal through all
body "Solid1"
